Autodesk Fusion 360 part; units mm, degrees
(part 2 of 4)
  spline S203 degree 2 poles (-3.5776, -2.4093) (-3.5776, -2.6712) (-3.7686, -2.854) knots 0 0 0 1 1 1
  spline S204 degree 2 poles (-3.7686, -2.854) (-3.9596, -3.0355) (-4.2515, -3.0355) knots 0 0 0 1 1 1
  spline S205 degree 2 poles (-4.2515, -3.0355) (-4.5148, -3.0355) (-4.6894, -2.8786) knots 0 0 0 1 1 1
  spline S206 degree 2 poles (-4.6894, -2.8786) (-4.8627, -2.7217) (-4.8872, -2.472) knots 0 0 0 1 1 1
  line L129 (-3.2351, -3) -> (-3.2351, -1)
  line L130 (-3.2351, -1) -> (-2.5462, -1)
  spline S207 degree 2 poles (-2.5462, -1) (-2.3129, -1) (-2.1901, -1.0286) knots 0 0 0 1 1 1
  spline S208 degree 2 poles (-2.1901, -1.0286) (-2.0182, -1.0682) (-1.8968, -1.1719) knots 0 0 0 1 1 1
  spline S209 degree 2 poles (-1.8968, -1.1719) (-1.7385, -1.3056) (-1.6608, -1.5143) knots 0 0 0 1 1 1
  spline S210 degree 2 poles (-1.6608, -1.5143) (-1.5817, -1.7217) (-1.5817, -1.9891) knots 0 0 0 1 1 1
  spline S211 degree 2 poles (-1.5817, -1.9891) (-1.5817, -2.2169) (-1.6349, -2.3929) knots 0 0 0 1 1 1
  spline S212 degree 2 poles (-1.6349, -2.3929) (-1.6881, -2.5689) (-1.7713, -2.6849) knots 0 0 0 1 1 1
  spline S213 degree 2 poles (-1.7713, -2.6849) (-1.8545, -2.7995) (-1.9541, -2.8663) knots 0 0 0 1 1 1
  spline S214 degree 2 poles (-1.9541, -2.8663) (-2.0523, -2.9318) (-2.1928, -2.9659) knots 0 0 0 1 1 1
  spline S215 degree 2 poles (-2.1928, -2.9659) (-2.332, -3) (-2.5134, -3) knots 0 0 0 1 1 1
  line L131 (-2.5134, -3) -> (-3.2351, -3)
  line L132 (-2.9705, -2.764) -> (-2.5435, -2.764)
  spline S216 degree 2 poles (-2.5435, -2.764) (-2.3456, -2.764) (-2.2338, -2.7271) knots 0 0 0 1 1 1
  spline S217 degree 2 poles (-2.2338, -2.7271) (-2.1205, -2.6903) (-2.0537, -2.6235) knots 0 0 0 1 1 1
  spline S218 degree 2 poles (-2.0537, -2.6235) (-1.9596, -2.5293) (-1.9077, -2.3711) knots 0 0 0 1 1 1
  spline S219 degree 2 poles (-1.9077, -2.3711) (-1.8545, -2.2115) (-1.8545, -1.985) knots 0 0 0 1 1 1
  spline S220 degree 2 poles (-1.8545, -1.985) (-1.8545, -1.6712) (-1.9582, -1.5034) knots 0 0 0 1 1 1
  spline S221 degree 2 poles (-1.9582, -1.5034) (-2.0605, -1.3342) (-2.2078, -1.2769) knots 0 0 0 1 1 1
  spline S222 degree 2 poles (-2.2078, -1.2769) (-2.3143, -1.236) (-2.5503, -1.236) knots 0 0 0 1 1 1
  line L133 (-2.5503, -1.236) -> (-2.9705, -1.236)
  line L134 (-2.9705, -1.236) -> (-2.9705, -2.764)
  line L135 (-0.5298, -3) -> (-0.5298, -2.5211)
  line L136 (-0.5298, -2.5211) -> (-1.3975, -2.5211)
  line L137 (-1.3975, -2.5211) -> (-1.3975, -2.296)
  line L138 (-1.3975, -2.296) -> (-0.4848, -1)
  line L139 (-0.4848, -1) -> (-0.2842, -1)
  line L140 (-0.2842, -1) -> (-0.2842, -2.296)
  line L141 (-0.2842, -2.296) -> (-0.0141, -2.296)
  line L142 (-0.0141, -2.296) -> (-0.0141, -2.5211)
  line L143 (-0.0141, -2.5211) -> (-0.2842, -2.5211)
  line L144 (-0.2842, -2.5211) -> (-0.2842, -3)
  line L145 (-0.2842, -3) -> (-0.5298, -3)
  line L146 (-0.5298, -2.296) -> (-0.5298, -1.3943)
  line L147 (-0.5298, -1.3943) -> (-1.156, -2.296)
  line L148 (-1.156, -2.296) -> (-0.5298, -2.296)
  line L149 (0.2096, -2.3997) -> (0.2096, -2.1528)
  line L150 (0.2096, -2.1528) -> (0.964, -2.1528)
  line L151 (0.964, -2.1528) -> (0.964, -2.3997)
  line L152 (0.964, -2.3997) -> (0.2096, -2.3997)
  line L153 (1.1769, -2.3574) -> (1.4265, -2.3356)
  spline S223 degree 2 poles (1.4265, -2.3356) (1.4443, -2.4857) (1.5084, -2.5825) knots 0 0 0 1 1 1
  spline S224 degree 2 poles (1.5084, -2.5825) (1.5739, -2.678) (1.7103, -2.7381) knots 0 0 0 1 1 1
  spline S225 degree 2 poles (1.7103, -2.7381) (1.8467, -2.7967) (2.0173, -2.7967) knots 0 0 0 1 1 1
  spline S226 degree 2 poles (2.0173, -2.7967) (2.1687, -2.7967) (2.2847, -2.7517) knots 0 0 0 1 1 1
  spline S227 degree 2 poles (2.2847, -2.7517) (2.4006, -2.7067) (2.4565, -2.6289) knots 0 0 0 1 1 1
  spline S228 degree 2 poles (2.4565, -2.6289) (2.5138, -2.5498) (2.5138, -2.457) knots 0 0 0 1 1 1
  spline S229 degree 2 poles (2.5138, -2.457) (2.5138, -2.3629) (2.4593, -2.2933) knots 0 0 0 1 1 1
  spline S230 degree 2 poles (2.4593, -2.2933) (2.4047, -2.2224) (2.2792, -2.1746) knots 0 0 0 1 1 1
  spline S231 degree 2 poles (2.2792, -2.1746) (2.1987, -2.1432) (1.9231, -2.0778) knots 0 0 0 1 1 1
  spline S232 degree 2 poles (1.9231, -2.0778) (1.6475, -2.0109) (1.537, -1.9523) knots 0 0 0 1 1 1
  spline S233 degree 2 poles (1.537, -1.9523) (1.3938, -1.8772) (1.3229, -1.7667) knots 0 0 0 1 1 1
  spline S234 degree 2 poles (1.3229, -1.7667) (1.2533, -1.6548) (1.2533, -1.5171) knots 0 0 0 1 1 1
  spline S235 degree 2 poles (1.2533, -1.5171) (1.2533, -1.3656) (1.3392, -1.2347) knots 0 0 0 1 1 1
  spline S236 degree 2 poles (1.3392, -1.2347) (1.4252, -1.1023) (1.5902, -1.0341) knots 0 0 0 1 1 1
  spline S237 degree 2 poles (1.5902, -1.0341) (1.7553, -0.9659) (1.9572, -0.9659) knots 0 0 0 1 1 1
  spline S238 degree 2 poles (1.9572, -0.9659) (2.1796, -0.9659) (2.3488, -1.0382) knots 0 0 0 1 1 1
  spline S239 degree 2 poles (2.3488, -1.0382) (2.5193, -1.1091) (2.6107, -1.2483) knots 0 0 0 1 1 1
  spline S240 degree 2 poles (2.6107, -1.2483) (2.7021, -1.3874) (2.7089, -1.5634) knots 0 0 0 1 1 1
  line L154 (2.7089, -1.5634) -> (2.4552, -1.5825)
  spline S241 degree 2 poles (2.4552, -1.5825) (2.4347, -1.3929) (2.316, -1.296) knots 0 0 0 1 1 1
  spline S242 degree 2 poles (2.316, -1.296) (2.1987, -1.1992) (1.9681, -1.1992) knots 0 0 0 1 1 1
  spline S243 degree 2 poles (1.9681, -1.1992) (1.728, -1.1992) (1.6175, -1.2879) knots 0 0 0 1 1 1
  spline S244 degree 2 poles (1.6175, -1.2879) (1.5084, -1.3752) (1.5084, -1.4993) knots 0 0 0 1 1 1
  spline S245 degree 2 poles (1.5084, -1.4993) (1.5084, -1.6071) (1.5862, -1.6767) knots 0 0 0 1 1 1
  spline S246 degree 2 poles (1.5862, -1.6767) (1.6626, -1.7462) (1.9845, -1.8199) knots 0 0 0 1 1 1
  spline S247 degree 2 poles (1.9845, -1.8199) (2.3078, -1.8922) (2.4279, -1.9468) knots 0 0 0 1 1 1
  spline S248 degree 2 poles (2.4279, -1.9468) (2.6025, -2.0273) (2.6857, -2.1514) knots 0 0 0 1 1 1
  spline S249 degree 2 poles (2.6857, -2.1514) (2.769, -2.2742) (2.769, -2.4352) knots 0 0 0 1 1 1
  spline S250 degree 2 poles (2.769, -2.4352) (2.769, -2.5948) (2.6776, -2.7367) knots 0 0 0 1 1 1
  spline S251 degree 2 poles (2.6776, -2.7367) (2.5862, -2.8772) (2.4143, -2.9563) knots 0 0 0 1 1 1
  spline S252 degree 2 poles (2.4143, -2.9563) (2.2437, -3.0341) (2.0295, -3.0341) knots 0 0 0 1 1 1
  spline S253 degree 2 poles (2.0295, -3.0341) (1.758, -3.0341) (1.5739, -2.955) knots 0 0 0 1 1 1
  spline S254 degree 2 poles (1.5739, -2.955) (1.3911, -2.8759) (1.286, -2.7176) knots 0 0 0 1 1 1
  spline S255 degree 2 poles (1.286, -2.7176) (1.1823, -2.558) (1.1769, -2.3574) knots 0 0 0 1 1 1
  line L155 (3.1305, -3) -> (3.1305, -1)
  line L156 (3.1305, -1) -> (3.8194, -1)
  spline S256 degree 2 poles (3.8194, -1) (4.0527, -1) (4.1755, -1.0286) knots 0 0 0 1 1 1
  spline S257 degree 2 poles (4.1755, -1.0286) (4.3474, -1.0682) (4.4688, -1.1719) knots 0 0 0 1 1 1
  spline S258 degree 2 poles (4.4688, -1.1719) (4.6271, -1.3056) (4.7048, -1.5143) knots 0 0 0 1 1 1
  spline S259 degree 2 poles (4.7048, -1.5143) (4.784, -1.7217) (4.784, -1.9891) knots 0 0 0 1 1 1
  spline S260 degree 2 poles (4.784, -1.9891) (4.784, -2.2169) (4.7308, -2.3929) knots 0 0 0 1 1 1
  spline S261 degree 2 poles (4.7308, -2.3929) (4.6776, -2.5689) (4.5943, -2.6849) knots 0 0 0 1 1 1
  spline S262 degree 2 poles (4.5943, -2.6849) (4.5111, -2.7995) (4.4115, -2.8663) knots 0 0 0 1 1 1
  spline S263 degree 2 poles (4.4115, -2.8663) (4.3133, -2.9318) (4.1728, -2.9659) knots 0 0 0 1 1 1
  spline S264 degree 2 poles (4.1728, -2.9659) (4.0336, -3) (3.8522, -3) knots 0 0 0 1 1 1
  line L157 (3.8522, -3) -> (3.1305, -3)
  line L158 (3.3952, -2.764) -> (3.8222, -2.764)
  spline S265 degree 2 poles (3.8222, -2.764) (4.02, -2.764) (4.1319, -2.7271) knots 0 0 0 1 1 1
  spline S266 degree 2 poles (4.1319, -2.7271) (4.2451, -2.6903) (4.3119, -2.6235) knots 0 0 0 1 1 1
  spline S267 degree 2 poles (4.3119, -2.6235) (4.4061, -2.5293) (4.4579, -2.3711) knots 0 0 0 1 1 1
  spline S268 degree 2 poles (4.4579, -2.3711) (4.5111, -2.2115) (4.5111, -1.985) knots 0 0 0 1 1 1
  spline S269 degree 2 poles (4.5111, -1.985) (4.5111, -1.6712) (4.4074, -1.5034) knots 0 0 0 1 1 1
  spline S270 degree 2 poles (4.4074, -1.5034) (4.3051, -1.3342) (4.1578, -1.2769) knots 0 0 0 1 1 1
  spline S271 degree 2 poles (4.1578, -1.2769) (4.0514, -1.236) (3.8153, -1.236) knots 0 0 0 1 1 1
  line L159 (3.8153, -1.236) -> (3.3952, -1.236)
  line L160 (3.3952, -1.236) -> (3.3952, -2.764)
  spline S272 degree 2 poles (5.5862, -3.588) (5.3829, -3.3315) (5.2424, -2.9877) knots 0 0 0 1 1 1
  spline S273 degree 2 poles (5.2424, -2.9877) (5.1018, -2.6439) (5.1018, -2.2756) knots 0 0 0 1 1 1
  spline S274 degree 2 poles (5.1018, -2.2756) (5.1018, -1.9509) (5.2069, -1.6535) knots 0 0 0 1 1 1
  spline S275 degree 2 poles (5.2069, -1.6535) (5.3297, -1.3083) (5.5862, -0.9659) knots 0 0 0 1 1 1
  line L161 (5.5862, -0.9659) -> (5.7621, -0.9659)
  spline S276 degree 2 poles (5.7621, -0.9659) (5.5971, -1.2497) (5.5439, -1.3711) knots 0 0 0 1 1 1
  spline S277 degree 2 poles (5.5439, -1.3711) (5.4606, -1.5593) (5.4129, -1.764) knots 0 0 0 1 1 1
  spline S278 degree 2 poles (5.4129, -1.764) (5.3542, -2.0191) (5.3542, -2.2769) knots 0 0 0 1 1 1
  spline S279 degree 2 poles (5.3542, -2.2769) (5.3542, -2.9332) (5.7621, -3.588) knots 0 0 0 1 1 1
  line L162 (5.7621, -3.588) -> (5.5862, -3.588)
  line L163 (6.904, -3) -> (6.6585, -3)
  line L164 (6.6585, -3) -> (6.6585, -1.4352)
  spline S280 degree 2 poles (6.6585, -1.4352) (6.5698, -1.5198) (6.4252, -1.6044) knots 0 0 0 1 1 1
  spline S281 degree 2 poles (6.4252, -1.6044) (6.2819, -1.6889) (6.1673, -1.7312) knots 0 0 0 1 1 1
  line L165 (6.1673, -1.7312) -> (6.1673, -1.4939)
  spline S282 degree 2 poles (6.1673, -1.4939) (6.3733, -1.397) (6.5275, -1.2592) knots 0 0 0 1 1 1
  spline S283 degree 2 poles (6.5275, -1.2592) (6.6816, -1.1214) (6.7458, -0.9918) knots 0 0 0 1 1 1
  line L166 (6.7458, -0.9918) -> (6.904, -0.9918)
  line L167 (6.904, -0.9918) -> (6.904, -3)
  line L168 (7.5329, -2.4761) -> (7.7908, -2.4543)
  spline S284 degree 2 poles (7.7908, -2.4543) (7.8194, -2.6426) (7.9231, -2.7381) knots 0 0 0 1 1 1
  spline S285 degree 2 poles (7.9231, -2.7381) (8.0282, -2.8322) (8.1755, -2.8322) knots 0 0 0 1 1 1
  spline S286 degree 2 poles (8.1755, -2.8322) (8.3529, -2.8322) (8.4756, -2.6985) knots 0 0 0 1 1 1
  spline S287 degree 2 poles (8.4756, -2.6985) (8.5984, -2.5648) (8.5984, -2.3438) knots 0 0 0 1 1 1
  spline S288 degree 2 poles (8.5984, -2.3438) (8.5984, -2.1337) (8.4797, -2.0123) knots 0 0 0 1 1 1
  spline S289 degree 2 poles (8.4797, -2.0123) (8.3624, -1.8909) (8.1714, -1.8909) knots 0 0 0 1 1 1
  spline S290 degree 2 poles (8.1714, -1.8909) (8.0527, -1.8909) (7.9572, -1.9454) knots 0 0 0 1 1 1
  spline S291 degree 2 poles (7.9572, -1.9454) (7.8617, -1.9986) (7.8072, -2.0846) knots 0 0 0 1 1 1
  line L169 (7.8072, -2.0846) -> (7.5766, -2.0546)
  line L170 (7.5766, -2.0546) -> (7.7703, -1.0273)
  line L171 (7.7703, -1.0273) -> (8.7649, -1.0273)
  line L172 (8.7649, -1.0273) -> (8.7649, -1.2619)
  line L173 (8.7649, -1.2619) -> (7.9668, -1.2619)
  line L174 (7.9668, -1.2619) -> (7.859, -1.7995)
  spline S292 degree 2 poles (7.859, -1.7995) (8.0391, -1.6739) (8.2369, -1.6739) knots 0 0 0 1 1 1
  spline S293 degree 2 poles (8.2369, -1.6739) (8.4988, -1.6739) (8.6789, -1.8554) knots 0 0 0 1 1 1
  spline S294 degree 2 poles (8.6789, -1.8554) (8.859, -2.0368) (8.859, -2.322) knots 0 0 0 1 1 1
  spline S295 degree 2 poles (8.859, -2.322) (8.859, -2.5935) (8.7007, -2.7913) knots 0 0 0 1 1 1
  spline S296 degree 2 poles (8.7007, -2.7913) (8.5084, -3.0341) (8.1755, -3.0341) knots 0 0 0 1 1 1
  spline S297 degree 2 poles (8.1755, -3.0341) (7.9027, -3.0341) (7.7294, -2.8813) knots 0 0 0 1 1 1
  spline S298 degree 2 poles (7.7294, -2.8813) (7.5575, -2.7285) (7.5329, -2.4761) knots 0 0 0 1 1 1
  line L175 (9.1032, -1.2619) -> (9.1032, -1.0259)
  line L176 (9.1032, -1.0259) -> (10.3979, -1.0259)
  line L177 (10.3979, -1.0259) -> (10.3979, -1.2169)
  spline S299 degree 2 poles (10.3979, -1.2169) (10.2069, -1.4202) (10.0186, -1.7572) knots 0 0 0 1 1 1
  spline S300 degree 2 poles (10.0186, -1.7572) (9.8317, -2.0941) (9.7294, -2.4502) knots 0 0 0 1 1 1
  spline S301 degree 2 poles (9.7294, -2.4502) (9.6557, -2.7012) (9.6353, -3) knots 0 0 0 1 1 1
  line L178 (9.6353, -3) -> (9.3829, -3)
  spline S302 degree 2 poles (9.3829, -3) (9.387, -2.764) (9.4756, -2.4297) knots 0 0 0 1 1 1
  spline S303 degree 2 poles (9.4756, -2.4297) (9.5643, -2.0955) (9.7294, -1.7858) knots 0 0 0 1 1 1
  spline S304 degree 2 poles (9.7294, -1.7858) (9.8958, -1.4748) (10.0827, -1.2619) knots 0 0 0 1 1 1
  line L179 (10.0827, -1.2619) -> (9.1032, -1.2619)
  line L180 (10.8699, -3.588) -> (10.6939, -3.588)
  spline S305 degree 2 poles (10.6939, -3.588) (11.1018, -2.9332) (11.1018, -2.2769) knots 0 0 0 1 1 1
  spline S306 degree 2 poles (11.1018, -2.2769) (11.1018, -2.0205) (11.0432, -1.7681) knots 0 0 0 1 1 1
  spline S307 degree 2 poles (11.0432, -1.7681) (10.9968, -1.5634) (10.9136, -1.3752) knots 0 0 0 1 1 1
  spline S308 degree 2 poles (10.9136, -1.3752) (10.8604, -1.2524) (10.6939, -0.9659) knots 0 0 0 1 1 1
  line L181 (10.6939, -0.9659) -> (10.8699, -0.9659)
  spline S309 degree 2 poles (10.8699, -0.9659) (11.1264, -1.3083) (11.2492, -1.6535) knots 0 0 0 1 1 1
  spline S310 degree 2 poles (11.2492, -1.6535) (11.3542, -1.9509) (11.3542, -2.2756) knots 0 0 0 1 1 1
  spline S311 degree 2 poles (11.3542, -2.2756) (11.3542, -2.6439) (11.2123, -2.9877) knots 0 0 0 1 1 1
  spline S312 degree 2 poles (11.2123, -2.9877) (11.0718, -3.3315) (10.8699, -3.588) knots 0 0 0 1 1 1
  spline S313 degree 2 poles (-11.8245, 0.9689) (-11.8245, 1.5664) (-11.5036, 1.9037) knots 0 0 0 1 1 1
  spline S314 degree 2 poles (-11.5036, 1.9037) (-11.1827, 2.2426) (-10.6752, 2.2426) knots 0 0 0 1 1 1
  spline S315 degree 2 poles (-10.6752, 2.2426) (-10.3429, 2.2426) (-10.0761, 2.0838) knots 0 0 0 1 1 1
  spline S316 degree 2 poles (-10.0761, 2.0838) (-9.8092, 1.925) (-9.6701, 1.6401) knots 0 0 0 1 1 1
  spline S317 degree 2 poles (-9.6701, 1.6401) (-9.5293, 1.3569) (-9.5293, 0.9967) knots 0 0 0 1 1 1
  spline S318 degree 2 poles (-9.5293, 0.9967) (-9.5293, 0.6317) (-9.6766, 0.3435) knots 0 0 0 1 1 1
  spline S319 degree 2 poles (-9.6766, 0.3435) (-9.8239, 0.0554) (-10.0941, -0.0936) knots 0 0 0 1 1 1
  spline S320 degree 2 poles (-10.0941, -0.0936) (-10.3642, -0.2409) (-10.6769, -0.2409) knots 0 0 0 1 1 1
  spline S321 degree 2 poles (-10.6769, -0.2409) (-11.0158, -0.2409) (-11.2826, -0.0772) knots 0 0 0 1 1 1
  spline S322 degree 2 poles (-11.2826, -0.0772) (-11.5495, 0.0865) (-11.687, 0.3697) knots 0 0 0 1 1 1
  spline S323 degree 2 poles (-11.687, 0.3697) (-11.8245, 0.6529) (-11.8245, 0.9689) knots 0 0 0 1 1 1
  spline S324 degree 2 poles (-11.4971, 0.964) (-11.4971, 0.5302) (-11.2646, 0.2797) knots 0 0 0 1 1 1
  spline S325 degree 2 poles (-11.2646, 0.2797) (-11.0305, 0.0308) (-10.6785, 0.0308) knots 0 0 0 1 1 1
  spline S326 degree 2 poles (-10.6785, 0.0308) (-10.32, 0.0308) (-10.0892, 0.2829) knots 0 0 0 1 1 1
  spline S327 degree 2 poles (-10.0892, 0.2829) (-9.8567, 0.5351) (-9.8567, 0.9984) knots 0 0 0 1 1 1
  spline S328 degree 2 poles (-9.8567, 0.9984) (-9.8567, 1.2914) (-9.9565, 1.5091) knots 0 0 0 1 1 1
  spline S329 degree 2 poles (-9.9565, 1.5091) (-10.0548, 1.7285) (-10.2463, 1.848) knots 0 0 0 1 1 1
  spline S330 degree 2 poles (-10.2463, 1.848) (-10.4362, 1.9692) (-10.6736, 1.9692) knots 0 0 0 1 1 1
  spline S331 degree 2 poles (-10.6736, 1.9692) (-11.0108, 1.9692) (-11.2548, 1.7367) knots 0 0 0 1 1 1
  spline S332 degree 2 poles (-11.2548, 1.7367) (-11.4971, 1.5059) (-11.4971, 0.964) knots 0 0 0 1 1 1
  line L182 (-8.8816, -0.2) -> (-8.8816, 2.2)
  line L183 (-8.8816, 2.2) -> (-7.9812, 2.2)
  spline S333 degree 2 poles (-7.9812, 2.2) (-7.7062, 2.2) (-7.5408, 2.1263) knots 0 0 0 1 1 1
  spline S334 degree 2 poles (-7.5408, 2.1263) (-7.3738, 2.0543) (-7.2805, 1.902) knots 0 0 0 1 1 1
  spline S335 degree 2 poles (-7.2805, 1.902) (-7.1856, 1.7514) (-7.1856, 1.5861) knots 0 0 0 1 1 1
  spline S336 degree 2 poles (-7.1856, 1.5861) (-7.1856, 1.4322) (-7.2691, 1.2963) knots 0 0 0 1 1 1
  spline S337 degree 2 poles (-7.2691, 1.2963) (-7.3526, 1.1604) (-7.5212, 1.0769) knots 0 0 0 1 1 1
  spline S338 degree 2 poles (-7.5212, 1.0769) (-7.3035, 1.0131) (-7.1872, 0.8592) knots 0 0 0 1 1 1
  spline S339 degree 2 poles (-7.1872, 0.8592) (-7.0693, 0.7053) (-7.0693, 0.4958) knots 0 0 0 1 1 1
  spline S340 degree 2 poles (-7.0693, 0.4958) (-7.0693, 0.3271) (-7.1414, 0.1814) knots 0 0 0 1 1 1
  spline S341 degree 2 poles (-7.1414, 0.1814) (-7.2118, 0.0374) (-7.3165, -0.0412) knots 0 0 0 1 1 1
  spline S342 degree 2 poles (-7.3165, -0.0412) (-7.4213, -0.1198) (-7.5801, -0.1607) knots 0 0 0 1 1 1
  spline S343 degree 2 poles (-7.5801, -0.1607) (-7.7373, -0.2) (-7.9665, -0.2) knots 0 0 0 1 1 1
  line L184 (-7.9665, -0.2) -> (-8.8816, -0.2)
  line L185 (-8.564, 1.1915) -> (-8.0451, 1.1915)
  spline S344 degree 2 poles (-8.0451, 1.1915) (-7.8339, 1.1915) (-7.7422, 1.2194) knots 0 0 0 1 1 1
  spline S345 degree 2 poles (-7.7422, 1.2194) (-7.6211, 1.2554) (-7.5605, 1.3389) knots 0 0 0 1 1 1
  spline S346 degree 2 poles (-7.5605, 1.3389) (-7.4983, 1.4224) (-7.4983, 1.5484) knots 0 0 0 1 1 1
  spline S347 degree 2 poles (-7.4983, 1.5484) (-7.4983, 1.6679) (-7.5556, 1.758) knots 0 0 0 1 1 1
  spline S348 degree 2 poles (-7.5556, 1.758) (-7.6129, 1.8497) (-7.7193, 1.8824) knots 0 0 0 1 1 1
  spline S349 degree 2 poles (-7.7193, 1.8824) (-7.8257, 1.9168) (-8.0844, 1.9168) knots 0 0 0 1 1 1
  line L186 (-8.0844, 1.9168) -> (-8.564, 1.9168)
  line L187 (-8.564, 1.9168) -> (-8.564, 1.1915)
  line L188 (-8.564, 0.0832) -> (-7.9665, 0.0832)
  spline S350 degree 2 poles (-7.9665, 0.0832) (-7.8126, 0.0832) (-7.7504, 0.0947) knots 0 0 0 1 1 1
  spline S351 degree 2 poles (-7.7504, 0.0947) (-7.6407, 0.1143) (-7.567, 0.1602) knots 0 0 0 1 1 1
  spline S352 degree 2 poles (-7.567, 0.1602) (-7.4934, 0.206) (-7.4459, 0.2928) knots 0 0 0 1 1 1
  spline S353 degree 2 poles (-7.4459, 0.2928) (-7.3984, 0.3812) (-7.3984, 0.4958) knots 0 0 0 1 1 1
  spline S354 degree 2 poles (-7.3984, 0.4958) (-7.3984, 0.63) (-7.4672, 0.7282) knots 0 0 0 1 1 1
  spline S355 degree 2 poles (-7.4672, 0.7282) (-7.5359, 0.8281) (-7.6587, 0.8674) knots 0 0 0 1 1 1
  spline S356 degree 2 poles (-7.6587, 0.8674) (-7.7799, 0.9083) (-8.009, 0.9083) knots 0 0 0 1 1 1
  line L189 (-8.009, 0.9083) -> (-8.564, 0.9083)
  line L190 (-8.564, 0.9083) -> (-8.564, 0.0832)
  line L191 (-6.4888, 0.5711) -> (-6.1892, 0.5973)
  spline S357 degree 2 poles (-6.1892, 0.5973) (-6.168, 0.4172) (-6.091, 0.301) knots 0 0 0 1 1 1
  spline S358 degree 2 poles (-6.091, 0.301) (-6.0124, 0.1864) (-5.8487, 0.1143) knots 0 0 0 1 1 1
  spline S359 degree 2 poles (-5.8487, 0.1143) (-5.685, 0.0439) (-5.4804, 0.0439) knots 0 0 0 1 1 1
  spline S360 degree 2 poles (-5.4804, 0.0439) (-5.2987, 0.0439) (-5.1595, 0.098) knots 0 0 0 1 1 1
  spline S361 degree 2 poles (-5.1595, 0.098) (-5.0203, 0.152) (-4.9532, 0.2453) knots 0 0 0 1 1 1
  spline S362 degree 2 poles (-4.9532, 0.2453) (-4.8845, 0.3402) (-4.8845, 0.4516) knots 0 0 0 1 1 1
  spline S363 degree 2 poles (-4.8845, 0.4516) (-4.8845, 0.5645) (-4.9499, 0.648) knots 0 0 0 1 1 1
  spline S364 degree 2 poles (-4.9499, 0.648) (-5.0154, 0.7332) (-5.166, 0.7905) knots 0 0 0 1 1 1
  spline S365 degree 2 poles (-5.166, 0.7905) (-5.2626, 0.8281) (-5.5933, 0.9067) knots 0 0 0 1 1 1
  spline S366 degree 2 poles (-5.5933, 0.9067) (-5.924, 0.9869) (-6.0566, 1.0573) knots 0 0 0 1 1 1
  spline S367 degree 2 poles (-6.0566, 1.0573) (-6.2285, 1.1473) (-6.3137, 1.2799) knots 0 0 0 1 1 1
  spline S368 degree 2 poles (-6.3137, 1.2799) (-6.3971, 1.4142) (-6.3971, 1.5795) knots 0 0 0 1 1 1
  spline S369 degree 2 poles (-6.3971, 1.5795) (-6.3971, 1.7613) (-6.294, 1.9184) knots 0 0 0 1 1 1
  spline S370 degree 2 poles (-6.294, 1.9184) (-6.1909, 2.0772) (-5.9928, 2.1591) knots 0 0 0 1 1 1
  spline S371 degree 2 poles (-5.9928, 2.1591) (-5.7947, 2.2409) (-5.5524, 2.2409) knots 0 0 0 1 1 1
  spline S372 degree 2 poles (-5.5524, 2.2409) (-5.2856, 2.2409) (-5.0826, 2.1542) knots 0 0 0 1 1 1
  spline S373 degree 2 poles (-5.0826, 2.1542) (-4.8779, 2.069) (-4.7682, 1.902) knots 0 0 0 1 1 1
  spline S374 degree 2 poles (-4.7682, 1.902) (-4.6585, 1.7351) (-4.6504, 1.5239) knots 0 0 0 1 1 1
  line L192 (-4.6504, 1.5239) -> (-4.9549, 1.501)
  spline S375 degree 2 poles (-4.9549, 1.501) (-4.9794, 1.7285) (-5.1218, 1.8447) knots 0 0 0 1 1 1
  spline S376 degree 2 poles (-5.1218, 1.8447) (-5.2626, 1.961) (-5.5393, 1.961) knots 0 0 0 1 1 1
  spline S377 degree 2 poles (-5.5393, 1.961) (-5.8274, 1.961) (-5.96, 1.8546) knots 0 0 0 1 1 1
  spline S378 degree 2 poles (-5.96, 1.8546) (-6.091, 1.7498) (-6.091, 1.6008) knots 0 0 0 1 1 1
  spline S379 degree 2 poles (-6.091, 1.6008) (-6.091, 1.4715) (-5.9977, 1.388) knots 0 0 0 1 1 1
  spline S380 degree 2 poles (-5.9977, 1.388) (-5.906, 1.3045) (-5.5197, 1.2161) knots 0 0 0 1 1 1
  spline S381 degree 2 poles (-5.5197, 1.2161) (-5.1317, 1.1293) (-4.9876, 1.0638) knots 0 0 0 1 1 1
  spline S382 degree 2 poles (-4.9876, 1.0638) (-4.778, 0.9673) (-4.6782, 0.8183) knots 0 0 0 1 1 1
  spline S383 degree 2 poles (-4.6782, 0.8183) (-4.5783, 0.6709) (-4.5783, 0.4778) knots 0 0 0 1 1 1
  spline S384 degree 2 poles (-4.5783, 0.4778) (-4.5783, 0.2862) (-4.688, 0.116) knots 0 0 0 1 1 1
  spline S385 degree 2 poles (-4.688, 0.116) (-4.7977, -0.0527) (-5.004, -0.1476) knots 0 0 0 1 1 1
  spline S386 degree 2 poles (-5.004, -0.1476) (-5.2086, -0.2409) (-5.4656, -0.2409) knots 0 0 0 1 1 1
  spline S387 degree 2 poles (-5.4656, -0.2409) (-5.7914, -0.2409) (-6.0124, -0.146) knots 0 0 0 1 1 1
  spline S388 degree 2 poles (-6.0124, -0.146) (-6.2318, -0.051) (-6.3579, 0.1389) knots 0 0 0 1 1 1
  spline S389 degree 2 poles (-6.3579, 0.1389) (-6.4823, 0.3304) (-6.4888, 0.5711) knots 0 0 0 1 1 1
  line L193 (-4.1566, -0.2) -> (-3.2349, 2.2)
  line L194 (-3.2349, 2.2) -> (-2.8928, 2.2)
  line L195 (-2.8928, 2.2) -> (-1.9105, -0.2)
  line L196 (-1.9105, -0.2) -> (-2.2723, -0.2)
  line L197 (-2.2723, -0.2) -> (-2.5522, 0.5269)
  line L198 (-2.5522, 0.5269) -> (-3.5558, 0.5269)
  line L199 (-3.5558, 0.5269) -> (-3.8194, -0.2)
  line L200 (-3.8194, -0.2) -> (-4.1566, -0.2)
  line L201 (-3.4641, 0.7855) -> (-2.6505, 0.7855)
  line L202 (-2.6505, 0.7855) -> (-2.9009, 1.4502)
  spline S390 degree 2 poles (-2.9009, 1.4502) (-3.0155, 1.7531) (-3.0712, 1.9479) knots 0 0 0 1 1 1
  spline S391 degree 2 poles (-3.0712, 1.9479) (-3.117, 1.7171) (-3.2005, 1.4895) knots 0 0 0 1 1 1
  line L203 (-3.2005, 1.4895) -> (-3.4641, 0.7855)
  line L204 (-1.5575, 0.5203) -> (-1.5575, 0.8166)
  line L205 (-1.5575, 0.8166) -> (-0.6522, 0.8166)
  line L206 (-0.6522, 0.8166) -> (-0.6522, 0.5203)
  line L207 (-0.6522, 0.5203) -> (-1.5575, 0.5203)
  line L208 (-0.0504, -0.2) -> (-0.0504, 2.2)
  line L209 (-0.0504, 2.2) -> (0.2672, 2.2)
  line L210 (0.2672, 2.2) -> (0.2672, 0.0832)
  line L211 (0.2672, 0.0832) -> (1.4492, 0.0832)
  line L212 (1.4492, 0.0832) -> (1.4492, -0.2)
  line L213 (1.4492, -0.2) -> (-0.0504, -0.2)
  line L214 (2.0886, -0.2) -> (2.0886, 2.2)
  line L215 (2.0886, 2.2) -> (2.4062, 2.2)
  line L216 (2.4062, 2.2) -> (2.4062, 1.2145)
  line L217 (2.4062, 1.2145) -> (3.6537, 1.2145)
  line L218 (3.6537, 1.2145) -> (3.6537, 2.2)
  line L219 (3.6537, 2.2) -> (3.9713, 2.2)
  line L220 (3.9713, 2.2) -> (3.9713, -0.2)
  line L221 (3.9713, -0.2) -> (3.6537, -0.2)
  line L222 (3.6537, -0.2) -> (3.6537, 0.9312)
  line L223 (3.6537, 0.9312) -> (2.4062, 0.9312)
  line L224 (2.4062, 0.9312) -> (2.4062, -0.2)
  line L225 (2.4062, -0.2) -> (2.0886, -0.2)
  line L226 (4.6435, 0.5711) -> (4.9431, 0.5973)
  spline S392 degree 2 poles (4.9431, 0.5973) (4.9644, 0.4172) (5.0413, 0.301) knots 0 0 0 1 1 1
  spline S393 degree 2 poles (5.0413, 0.301) (5.1199, 0.1864) (5.2836, 0.1143) knots 0 0 0 1 1 1
  spline S394 degree 2 poles (5.2836, 0.1143) (5.4473, 0.0439) (5.652, 0.0439) knots 0 0 0 1 1 1
  spline S395 degree 2 poles (5.652, 0.0439) (5.8337, 0.0439) (5.9728, 0.098) knots 0 0 0 1 1 1
  spline S396 degree 2 poles (5.9728, 0.098) (6.112, 0.152) (6.1791, 0.2453) knots 0 0 0 1 1 1
  spline S397 degree 2 poles (6.1791, 0.2453) (6.2479, 0.3402) (6.2479, 0.4516) knots 0 0 0 1 1 1
  spline S398 degree 2 poles (6.2479, 0.4516) (6.2479, 0.5645) (6.1824, 0.648) knots 0 0 0 1 1 1
  spline S399 degree 2 poles (6.1824, 0.648) (6.1169, 0.7332) (5.9663, 0.7905) knots 0 0 0 1 1 1
  spline S400 degree 2 poles (5.9663, 0.7905) (5.8697, 0.8281) (5.539, 0.9067) knots 0 0 0 1 1 1
  spline S401 degree 2 poles (5.539, 0.9067) (5.2083, 0.9869) (5.0757, 1.0573) knots 0 0 0 1 1 1
  spline S402 degree 2 poles (5.0757, 1.0573) (4.9038, 1.1473) (4.8187, 1.2799) knots 0 0 0 1 1 1
  spline S403 degree 2 poles (4.8187, 1.2799) (4.7352, 1.4142) (4.7352, 1.5795) knots 0 0 0 1 1 1
  spline S404 degree 2 poles (4.7352, 1.5795) (4.7352, 1.7613) (4.8383, 1.9184) knots 0 0 0 1 1 1
  spline S405 degree 2 poles (4.8383, 1.9184) (4.9415, 2.0772) (5.1395, 2.1591) knots 0 0 0 1 1 1
  spline S406 degree 2 poles (5.1395, 2.1591) (5.3376, 2.2409) (5.5799, 2.2409) knots 0 0 0 1 1 1
  spline S407 degree 2 poles (5.5799, 2.2409) (5.8468, 2.2409) (6.0498, 2.1542) knots 0 0 0 1 1 1
  spline S408 degree 2 poles (6.0498, 2.1542) (6.2544, 2.069) (6.3641, 1.902) knots 0 0 0 1 1 1
  spline S409 degree 2 poles (6.3641, 1.902) (6.4738, 1.7351) (6.482, 1.5239) knots 0 0 0 1 1 1
  line L227 (6.482, 1.5239) -> (6.1775, 1.501)
  spline S410 degree 2 poles (6.1775, 1.501) (6.1529, 1.7285) (6.0105, 1.8447) knots 0 0 0 1 1 1
  spline S411 degree 2 poles (6.0105, 1.8447) (5.8697, 1.961) (5.593, 1.961) knots 0 0 0 1 1 1
  spline S412 degree 2 poles (5.593, 1.961) (5.3049, 1.961) (5.1723, 1.8546) knots 0 0 0 1 1 1
  spline S413 degree 2 poles (5.1723, 1.8546) (5.0413, 1.7498) (5.0413, 1.6008) knots 0 0 0 1 1 1
  spline S414 degree 2 poles (5.0413, 1.6008) (5.0413, 1.4715) (5.1346, 1.388) knots 0 0 0 1 1 1
  spline S415 degree 2 poles (5.1346, 1.388) (5.2263, 1.3045) (5.6127, 1.2161) knots 0 0 0 1 1 1
  spline S416 degree 2 poles (5.6127, 1.2161) (6.0007, 1.1293) (6.1447, 1.0638) knots 0 0 0 1 1 1
  spline S417 degree 2 poles (6.1447, 1.0638) (6.3543, 0.9673) (6.4541, 0.8183) knots 0 0 0 1 1 1
  spline S418 degree 2 poles (6.4541, 0.8183) (6.554, 0.6709) (6.554, 0.4778) knots 0 0 0 1 1 1
  spline S419 degree 2 poles (6.554, 0.4778) (6.554, 0.2862) (6.4443, 0.116) knots 0 0 0 1 1 1
  spline S420 degree 2 poles (6.4443, 0.116) (6.3346, -0.0527) (6.1284, -0.1476) knots 0 0 0 1 1 1
  spline S421 degree 2 poles (6.1284, -0.1476) (5.9237, -0.2409) (5.6667, -0.2409) knots 0 0 0 1 1 1
  spline S422 degree 2 poles (5.6667, -0.2409) (5.3409, -0.2409) (5.1199, -0.146) knots 0 0 0 1 1 1
  spline S423 degree 2 poles (5.1199, -0.146) (4.9005, -0.051) (4.7745, 0.1389) knots 0 0 0 1 1 1
  spline S424 degree 2 poles (4.7745, 0.1389) (4.6501, 0.3304) (4.6435, 0.5711) knots 0 0 0 1 1 1
  line L228 (8.2298, -0.2) -> (7.9351, -0.2)
  line L229 (7.9351, -0.2) -> (7.9351, 1.6778)
  spline S425 degree 2 poles (7.9351, 1.6778) (7.8287, 1.5763) (7.6551, 1.4748) knots 0 0 0 1 1 1
  spline S426 degree 2 poles (7.6551, 1.4748) (7.4832, 1.3733) (7.3457, 1.3225) knots 0 0 0 1 1 1
  line L230 (7.3457, 1.3225) -> (7.3457, 1.6074)
  spline S427 degree 2 poles (7.3457, 1.6074) (7.5929, 1.7236) (7.7779, 1.8889) knots 0 0 0 1 1 1
  spline S428 degree 2 poles (7.7779, 1.8889) (7.9629, 2.0543) (8.0398, 2.2098) knots 0 0 0 1 1 1
  line L231 (8.0398, 2.2098) -> (8.2298, 2.2098)
  line L232 (8.2298, 2.2098) -> (8.2298, -0.2)
  line L233 (9.3718, -0.2) -> (9.3718, 2.2)
  line L234 (9.3718, 2.2) -> (10.9909, 2.2)
  line L235 (10.9909, 2.2) -> (10.9909, 1.9168)
  line L236 (10.9909, 1.9168) -> (9.6894, 1.9168)
  line L237 (9.6894, 1.9168) -> (9.6894, 1.1735)
  line L238 (9.6894, 1.1735) -> (10.8157, 1.1735)
  line L239 (10.8157, 1.1735) -> (10.8157, 0.8903)
  line L240 (10.8157, 0.8903) -> (9.6894, 0.8903)
  line L241 (9.6894, 0.8903) -> (9.6894, -0.2)
  line L242 (9.6894, -0.2) -> (9.3718, -0.2)
  spline S429 degree 2 poles (-5.2607, -5.0136) (-5.2607, -4.6589) (-5.1884, -4.4434) knots 0 0 0 1 1 1
  spline S430 degree 2 poles (-5.1884, -4.4434) (-5.1148, -4.2265) (-4.9715, -4.1091) knots 0 0 0 1 1 1
  spline S431 degree 2 poles (-4.9715, -4.1091) (-4.8269, -3.9918) (-4.6086, -3.9918) knots 0 0 0 1 1 1
  spline S432 degree 2 poles (-4.6086, -3.9918) (-4.4476, -3.9918) (-4.3262, -4.0573) knots 0 0 0 1 1 1
  spline S433 degree 2 poles (-4.3262, -4.0573) (-4.2048, -4.1214) (-4.1257, -4.2442) knots 0 0 0 1 1 1
  spline S434 degree 2 poles (-4.1257, -4.2442) (-4.0466, -4.3656) (-4.0015, -4.5416) knots 0 0 0 1 1 1
  spline S435 degree 2 poles (-4.0015, -4.5416) (-3.9565, -4.7162) (-3.9565, -5.0136) knots 0 0 0 1 1 1
  spline S436 degree 2 poles (-3.9565, -5.0136) (-3.9565, -5.3656) (-4.0288, -5.5825) knots 0 0 0 1 1 1
  spline S437 degree 2 poles (-4.0288, -5.5825) (-4.1011, -5.7981) (-4.2457, -5.9168) knots 0 0 0 1 1 1
  spline S438 degree 2 poles (-4.2457, -5.9168) (-4.389, -6.0341) (-4.6086, -6.0341) knots 0 0 0 1 1 1
  spline S439 degree 2 poles (-4.6086, -6.0341) (-4.8979, -6.0341) (-5.0629, -5.8267) knots 0 0 0 1 1 1
  spline S440 degree 2 poles (-5.0629, -5.8267) (-5.2607, -5.5771) (-5.2607, -5.0136) knots 0 0 0 1 1 1
  spline S441 degree 2 poles (-5.0084, -5.0136) (-5.0084, -5.5061) (-4.8938, -5.6698) knots 0 0 0 1 1 1
  spline S442 degree 2 poles (-4.8938, -5.6698) (-4.7778, -5.8322) (-4.6086, -5.8322) knots 0 0 0 1 1 1
  spline S443 degree 2 poles (-4.6086, -5.8322) (-4.4395, -5.8322) (-4.3249, -5.6685) knots 0 0 0 1 1 1
  spline S444 degree 2 poles (-4.3249, -5.6685) (-4.2089, -5.5048) (-4.2089, -5.0136) knots 0 0 0 1 1 1
  spline S445 degree 2 poles (-4.2089, -5.0136) (-4.2089, -4.5198) (-4.3249, -4.3574) knots 0 0 0 1 1 1
  spline S446 degree 2 poles (-4.3249, -4.3574) (-4.4395, -4.1951) (-4.6114, -4.1951) knots 0 0 0 1 1 1
  spline S447 degree 2 poles (-4.6114, -4.1951) (-4.7805, -4.1951) (-4.8815, -4.3383) knots 0 0 0 1 1 1
  spline S448 degree 2 poles (-4.8815, -4.3383) (-5.0084, -4.5211) (-5.0084, -5.0136) knots 0 0 0 1 1 1
  line L243 (-3.5691, -6) -> (-3.5691, -5.7203)
  line L244 (-3.5691, -5.7203) -> (-3.2894, -5.7203)
  line L245 (-3.2894, -5.7203) -> (-3.2894, -6)
  line L246 (-3.2894, -6) -> (-3.5691, -6)
  line L247 (-2.0056, -6) -> (-2.2512, -6)
  line L248 (-2.2512, -6) -> (-2.2512, -4.4352)
  spline S449 degree 2 poles (-2.2512, -4.4352) (-2.3399, -4.5198) (-2.4845, -4.6044) knots 0 0 0 1 1 1
  spline S450 degree 2 poles (-2.4845, -4.6044) (-2.6277, -4.6889) (-2.7423, -4.7312) knots 0 0 0 1 1 1
  line L249 (-2.7423, -4.7312) -> (-2.7423, -4.4939)
  spline S451 degree 2 poles (-2.7423, -4.4939) (-2.5363, -4.397) (-2.3822, -4.2592) knots 0 0 0 1 1 1
  spline S452 degree 2 poles (-2.3822, -4.2592) (-2.228, -4.1214) (-2.1639, -3.9918) knots 0 0 0 1 1 1
  line L250 (-2.1639, -3.9918) -> (-2.0056, -3.9918)
  line L251 (-2.0056, -3.9918) -> (-2.0056, -6)
  line L252 (-1.4968, -6) -> (-0.7287, -4)
  line L253 (-0.7287, -4) -> (-0.4436, -4)
  line L254 (-0.4436, -4) -> (0.375, -6)
  line L255 (0.375, -6) -> (0.0735, -6)
  line L256 (0.0735, -6) -> (-0.1598, -5.3943)
  line L257 (-0.1598, -5.3943) -> (-0.9961, -5.3943)
  line L258 (-0.9961, -5.3943) -> (-1.2157, -6)
  line L259 (-1.2157, -6) -> (-1.4968, -6)
  line L260 (-0.9197, -5.1787) -> (-0.2416, -5.1787)
  line L261 (-0.2416, -5.1787) -> (-0.4504, -4.6248)
  spline S453 degree 2 poles (-0.4504, -4.6248) (-0.5459, -4.3724) (-0.5923, -4.2101) knots 0 0 0 1 1 1
  spline S454 degree 2 poles (-0.5923, -4.2101) (-0.6305, -4.4025) (-0.7, -4.5921) knots 0 0 0 1 1 1
  line L262 (-0.7, -4.5921) -> (-0.9197, -5.1787)
  line L263 (2.596, -5.472) -> (2.8416, -5.4393)
  spline S455 degree 2 poles (2.8416, -5.4393) (2.8839, -5.648) (2.9848, -5.7408) knots 0 0 0 1 1 1
  spline S456 degree 2 poles (2.9848, -5.7408) (3.0871, -5.8322) (3.2331, -5.8322) knots 0 0 0 1 1 1
  spline S457 degree 2 poles (3.2331, -5.8322) (3.4064, -5.8322) (3.5251, -5.7121) knots 0 0 0 1 1 1
  spline S458 degree 2 poles (3.5251, -5.7121) (3.6451, -5.5921) (3.6451, -5.4147) knots 0 0 0 1 1 1
  spline S459 degree 2 poles (3.6451, -5.4147) (3.6451, -5.2456) (3.5346, -5.1364) knots 0 0 0 1 1 1
  spline S460 degree 2 poles (3.5346, -5.1364) (3.4241, -5.0259) (3.2536, -5.0259) knots 0 0 0 1 1 1
  spline S461 degree 2 poles (3.2536, -5.0259) (3.184, -5.0259) (3.0803, -5.0532) knots 0 0 0 1 1 1
  line L264 (3.0803, -5.0532) -> (3.1076, -4.8377)
  spline S462 degree 2 poles (3.1076, -4.8377) (3.1322, -4.8404) (3.1472, -4.8404) knots 0 0 0 1 1 1
  spline S463 degree 2 poles (3.1472, -4.8404) (3.3041, -4.8404) (3.4296, -4.7585) knots 0 0 0 1 1 1
  spline S464 degree 2 poles (3.4296, -4.7585) (3.5551, -4.6767) (3.5551, -4.5061) knots 0 0 0 1 1 1
  spline S465 degree 2 poles (3.5551, -4.5061) (3.5551, -4.3711) (3.4637, -4.2824) knots 0 0 0 1 1 1
  spline S466 degree 2 poles (3.4637, -4.2824) (3.3723, -4.1937) (3.2277, -4.1937) knots 0 0 0 1 1 1
  spline S467 degree 2 poles (3.2277, -4.1937) (3.0844, -4.1937) (2.9889, -4.2838) knots 0 0 0 1 1 1
  spline S468 degree 2 poles (2.9889, -4.2838) (2.8934, -4.3738) (2.8661, -4.5539) knots 0 0 0 1 1 1
  line L265 (2.8661, -4.5539) -> (2.6206, -4.5102)
  spline S469 degree 2 poles (2.6206, -4.5102) (2.6656, -4.2633) (2.8252, -4.1282) knots 0 0 0 1 1 1
  spline S470 degree 2 poles (2.8252, -4.1282) (2.9848, -3.9918) (3.2222, -3.9918) knots 0 0 0 1 1 1
  spline S471 degree 2 poles (3.2222, -3.9918) (3.3859, -3.9918) (3.5237, -4.0628) knots 0 0 0 1 1 1
  spline S472 degree 2 poles (3.5237, -4.0628) (3.6615, -4.1323) (3.7338, -4.2538) knots 0 0 0 1 1 1
  spline S473 degree 2 poles (3.7338, -4.2538) (3.8075, -4.3752) (3.8075, -4.5116) knots 0 0 0 1 1 1
  spline S474 degree 2 poles (3.8075, -4.5116) (3.8075, -4.6412) (3.7379, -4.7476) knots 0 0 0 1 1 1
  spline S475 degree 2 poles (3.7379, -4.7476) (3.6683, -4.854) (3.5319, -4.9168) knots 0 0 0 1 1 1
  spline S476 degree 2 poles (3.5319, -4.9168) (3.7092, -4.9577) (3.8075, -5.0873) knots 0 0 0 1 1 1
  spline S477 degree 2 poles (3.8075, -5.0873) (3.9057, -5.2156) (3.9057, -5.4093) knots 0 0 0 1 1 1
  spline S478 degree 2 poles (3.9057, -5.4093) (3.9057, -5.6712) (3.7147, -5.854) knots 0 0 0 1 1 1
  spline S479 degree 2 poles (3.7147, -5.854) (3.5237, -6.0355) (3.2318, -6.0355) knots 0 0 0 1 1 1
  spline S480 degree 2 poles (3.2318, -6.0355) (2.9685, -6.0355) (2.7938, -5.8786) knots 0 0 0 1 1 1
  spline S481 degree 2 poles (2.7938, -5.8786) (2.6206, -5.7217) (2.596, -5.472) knots 0 0 0 1 1 1
  spline S482 degree 2 poles (4.1485, -5.0136) (4.1485, -4.6589) (4.2208, -4.4434) knots 0 0 0 1 1 1
  spline S483 degree 2 poles (4.2208, -4.4434) (4.2945, -4.2265) (4.4378, -4.1091) knots 0 0 0 1 1 1
  spline S484 degree 2 poles (4.4378, -4.1091) (4.5824, -3.9918) (4.8006, -3.9918) knots 0 0 0 1 1 1
  spline S485 degree 2 poles (4.8006, -3.9918) (4.9616, -3.9918) (5.083, -4.0573) knots 0 0 0 1 1 1
  spline S486 degree 2 poles (5.083, -4.0573) (5.2045, -4.1214) (5.2836, -4.2442) knots 0 0 0 1 1 1
  spline S487 degree 2 poles (5.2836, -4.2442) (5.3627, -4.3656) (5.4077, -4.5416) knots 0 0 0 1 1 1
  spline S488 degree 2 poles (5.4077, -4.5416) (5.4528, -4.7162) (5.4528, -5.0136) knots 0 0 0 1 1 1
  spline S489 degree 2 poles (5.4528, -5.0136) (5.4528, -5.3656) (5.3805, -5.5825) knots 0 0 0 1 1 1
  spline S490 degree 2 poles (5.3805, -5.5825) (5.3082, -5.7981) (5.1635, -5.9168) knots 0 0 0 1 1 1
  spline S491 degree 2 poles (5.1635, -5.9168) (5.0203, -6.0341) (4.8006, -6.0341) knots 0 0 0 1 1 1
  spline S492 degree 2 poles (4.8006, -6.0341) (4.5114, -6.0341) (4.3464, -5.8267) knots 0 0 0 1 1 1
  spline S493 degree 2 poles (4.3464, -5.8267) (4.1485, -5.5771) (4.1485, -5.0136) knots 0 0 0 1 1 1
  spline S494 degree 2 poles (4.4009, -5.0136) (4.4009, -5.5061) (4.5155, -5.6698) knots 0 0 0 1 1 1
  spline S495 degree 2 poles (4.5155, -5.6698) (4.6315, -5.8322) (4.8006, -5.8322) knots 0 0 0 1 1 1
  spline S496 degree 2 poles (4.8006, -5.8322) (4.9698, -5.8322) (5.0844, -5.6685) knots 0 0 0 1 1 1
  spline S497 degree 2 poles (5.0844, -5.6685) (5.2004, -5.5048) (5.2004, -5.0136) knots 0 0 0 1 1 1
  spline S498 degree 2 poles (5.2004, -5.0136) (5.2004, -4.5198) (5.0844, -4.3574) knots 0 0 0 1 1 1
  spline S499 degree 2 poles (5.0844, -4.3574) (4.9698, -4.1951) (4.7979, -4.1951) knots 0 0 0 1 1 1
  spline S500 degree 2 poles (4.7979, -4.1951) (4.6288, -4.1951) (4.5278, -4.3383) knots 0 0 0 1 1 1
  spline S501 degree 2 poles (4.5278, -4.3383) (4.4009, -4.5211) (4.4009, -5.0136) knots 0 0 0 1 1 1
  line L266 (6.3736, -6) -> (5.5987, -4)
  line L267 (5.5987, -4) -> (5.8852, -4)
  line L268 (5.8852, -4) -> (6.405, -5.4529)
  spline S502 degree 2 poles (6.405, -5.4529) (6.4678, -5.6276) (6.5101, -5.7804) knots 0 0 0 1 1 1
  spline S503 degree 2 poles (6.5101, -5.7804) (6.5564, -5.6166) (6.6178, -5.4529) knots 0 0 0 1 1 1
  line L269 (6.6178, -5.4529) -> (7.1581, -4)
  line L270 (7.1581, -4) -> (7.4282, -4)
  line L271 (7.4282, -4) -> (6.6451, -6)
  line L272 (6.6451, -6) -> (6.3736, -6)
  line L273 (7.6656, -6) -> (7.6656, -4)
  line L274 (7.6656, -4) -> (8.3545, -4)
  spline S504 degree 2 poles (8.3545, -4) (8.5878, -4) (8.7106, -4.0286) knots 0 0 0 1 1 1
  spline S505 degree 2 poles (8.7106, -4.0286) (8.8825, -4.0682) (9.0039, -4.1719) knots 0 0 0 1 1 1
  spline S506 degree 2 poles (9.0039, -4.1719) (9.1622, -4.3056) (9.2399, -4.5143) knots 0 0 0 1 1 1
  spline S507 degree 2 poles (9.2399, -4.5143) (9.3191, -4.7217) (9.3191, -4.9891) knots 0 0 0 1 1 1
  spline S508 degree 2 poles (9.3191, -4.9891) (9.3191, -5.2169) (9.2659, -5.3929) knots 0 0 0 1 1 1
  spline S509 degree 2 poles (9.2659, -5.3929) (9.2127, -5.5689) (9.1294, -5.6849) knots 0 0 0 1 1 1
  spline S510 degree 2 poles (9.1294, -5.6849) (9.0462, -5.7995) (8.9466, -5.8663) knots 0 0 0 1 1 1
  spline S511 degree 2 poles (8.9466, -5.8663) (8.8484, -5.9318) (8.7079, -5.9659) knots 0 0 0 1 1 1
  spline S512 degree 2 poles (8.7079, -5.9659) (8.5687, -6) (8.3873, -6) knots 0 0 0 1 1 1
  line L275 (8.3873, -6) -> (7.6656, -6)
  line L276 (7.9303, -5.764) -> (8.3573, -5.764)
  spline S513 degree 2 poles (8.3573, -5.764) (8.5551, -5.764) (8.667, -5.7271) knots 0 0 0 1 1 1
  spline S514 degree 2 poles (8.667, -5.7271) (8.7802, -5.6903) (8.847, -5.6235) knots 0 0 0 1 1 1
  spline S515 degree 2 poles (8.847, -5.6235) (8.9412, -5.5293) (8.993, -5.3711) knots 0 0 0 1 1 1
  spline S516 degree 2 poles (8.993, -5.3711) (9.0462, -5.2115) (9.0462, -4.985) knots 0 0 0 1 1 1
  spline S517 degree 2 poles (9.0462, -4.985) (9.0462, -4.6712) (8.9425, -4.5034) knots 0 0 0 1 1 1
  spline S518 degree 2 poles (8.9425, -4.5034) (8.8402, -4.3342) (8.6929, -4.2769) knots 0 0 0 1 1 1
  spline S519 degree 2 poles (8.6929, -4.2769) (8.5865, -4.236) (8.3504, -4.236) knots 0 0 0 1 1 1
  line L277 (8.3504, -4.236) -> (7.9303, -4.236)
  line L278 (7.9303, -4.236) -> (7.9303, -5.764)
  line L279 (11.1103, -5.2988) -> (11.375, -5.3656)
  spline S520 degree 2 poles (11.375, -5.3656) (11.2918, -5.6917) (11.0749, -5.8636) knots 0 0 0 1 1 1
  spline S521 degree 2 poles (11.0749, -5.8636) (10.8593, -6.0341) (10.5469, -6.0341) knots 0 0 0 1 1 1
  spline S522 degree 2 poles (10.5469, -6.0341) (10.2236, -6.0341) (10.0203, -5.9031) knots 0 0 0 1 1 1
  spline S523 degree 2 poles (10.0203, -5.9031) (9.8184, -5.7708) (9.712, -5.5211) knots 0 0 0 1 1 1
  spline S524 degree 2 poles (9.712, -5.5211) (9.6069, -5.2715) (9.6069, -4.985) knots 0 0 0 1 1 1
  spline S525 degree 2 poles (9.6069, -4.985) (9.6069, -4.6726) (9.7256, -4.4407) knots 0 0 0 1 1 1
  spline S526 degree 2 poles (9.7256, -4.4407) (9.8457, -4.2074) (10.0653, -4.0873) knots 0 0 0 1 1 1
  spline S527 degree 2 poles (10.0653, -4.0873) (10.2863, -3.9659) (10.551, -3.9659) knots 0 0 0 1 1 1
  spline S528 degree 2 poles (10.551, -3.9659) (10.8511, -3.9659) (11.0558, -4.1187) knots 0 0 0 1 1 1
  spline S529 degree 2 poles (11.0558, -4.1187) (11.2604, -4.2715) (11.3409, -4.5484) knots 0 0 0 1 1 1
  line L280 (11.3409, -4.5484) -> (11.0803, -4.6098)
  spline S530 degree 2 poles (11.0803, -4.6098) (11.0107, -4.3915) (10.8784, -4.292) knots 0 0 0 1 1 1
  spline S531 degree 2 poles (10.8784, -4.292) (10.7461, -4.1924) (10.5455, -4.1924) knots 0 0 0 1 1 1
  spline S532 degree 2 poles (10.5455, -4.1924) (10.315, -4.1924) (10.1594, -4.3029) knots 0 0 0 1 1 1
  spline S533 degree 2 poles (10.1594, -4.3029) (10.0053, -4.4134) (9.9425, -4.6003) knots 0 0 0 1 1 1
  spline S534 degree 2 poles (9.9425, -4.6003) (9.8798, -4.7858) (9.8798, -4.9836) knots 0 0 0 1 1 1
  spline S535 degree 2 poles (9.8798, -4.9836) (9.8798, -5.2387) (9.9534, -5.4297) knots 0 0 0 1 1 1
  spline S536 degree 2 poles (9.9534, -5.4297) (10.0285, -5.6194) (10.1854, -5.7135) knots 0 0 0 1 1 1
  spline S537 degree 2 poles (10.1854, -5.7135) (10.3423, -5.8076) (10.5251, -5.8076) knots 0 0 0 1 1 1
  spline S538 degree 2 poles (10.5251, -5.8076) (10.7474, -5.8076) (10.9016, -5.6794) knots 0 0 0 1 1 1
  spline S539 degree 2 poles (10.9016, -5.6794) (11.0558, -5.5512) (11.1103, -5.2988) knots 0 0 0 1 1 1
  spline S540 degree 2 poles (-11.2539, 3.9898) (-11.2539, 4.2558) (-11.1997, 4.4175) knots 0 0 0 1 1 1
  spline S541 degree 2 poles (-11.1997, 4.4175) (-11.1444, 4.5802) (-11.037, 4.6681) knots 0 0 0 1 1 1
  spline S542 degree 2 poles (-11.037, 4.6681) (-10.9285, 4.7561) (-10.7648, 4.7561) knots 0 0 0 1 1 1
  spline S543 degree 2 poles (-10.7648, 4.7561) (-10.6441, 4.7561) (-10.553, 4.707) knots 0 0 0 1 1 1
  spline S544 degree 2 poles (-10.553, 4.707) (-10.4619, 4.6589) (-10.4026, 4.5668) knots 0 0 0 1 1 1
  spline S545 degree 2 poles (-10.4026, 4.5668) (-10.3432, 4.4758) (-10.3095, 4.3438) knots 0 0 0 1 1 1
  spline S546 degree 2 poles (-10.3095, 4.3438) (-10.2757, 4.2128) (-10.2757, 3.9898) knots 0 0 0 1 1 1
  spline S547 degree 2 poles (-10.2757, 3.9898) (-10.2757, 3.7258) (-10.3299, 3.5631) knots 0 0 0 1 1 1
  spline S548 degree 2 poles (-10.3299, 3.5631) (-10.3842, 3.4014) (-10.4926, 3.3124) knots 0 0 0 1 1 1
  spline S549 degree 2 poles (-10.4926, 3.3124) (-10.6001, 3.2244) (-10.7648, 3.2244) knots 0 0 0 1 1 1
  spline S550 degree 2 poles (-10.7648, 3.2244) (-10.9817, 3.2244) (-11.1055, 3.3799) knots 0 0 0 1 1 1
  spline S551 degree 2 poles (-11.1055, 3.3799) (-11.2539, 3.5672) (-11.2539, 3.9898) knots 0 0 0 1 1 1
  spline S552 degree 2 poles (-11.0646, 3.9898) (-11.0646, 3.6204) (-10.9787, 3.4976) knots 0 0 0 1 1 1
  spline S553 degree 2 poles (-10.9787, 3.4976) (-10.8917, 3.3759) (-10.7648, 3.3759) knots 0 0 0 1 1 1
  spline S554 degree 2 poles (-10.7648, 3.3759) (-10.6379, 3.3759) (-10.552, 3.4986) knots 0 0 0 1 1 1
  spline S555 degree 2 poles (-10.552, 3.4986) (-10.465, 3.6214) (-10.465, 3.9898) knots 0 0 0 1 1 1
  spline S556 degree 2 poles (-10.465, 3.9898) (-10.465, 4.3602) (-10.552, 4.4819) knots 0 0 0 1 1 1
  spline S557 degree 2 poles (-10.552, 4.4819) (-10.6379, 4.6037) (-10.7669, 4.6037) knots 0 0 0 1 1 1
  spline S558 degree 2 poles (-10.7669, 4.6037) (-10.8937, 4.6037) (-10.9694, 4.4962) knots 0 0 0 1 1 1
  spline S559 degree 2 poles (-10.9694, 4.4962) (-11.0646, 4.3591) (-11.0646, 3.9898) knots 0 0 0 1 1 1
  line L281 (-10.0875, 3.646) -> (-9.9033, 3.6705)
  spline S560 degree 2 poles (-9.9033, 3.6705) (-9.8716, 3.514) (-9.7958, 3.4444) knots 0 0 0 1 1 1
  spline S561 degree 2 poles (-9.7958, 3.4444) (-9.7191, 3.3759) (-9.6096, 3.3759) knots 0 0 0 1 1 1
  spline S562 degree 2 poles (-9.6096, 3.3759) (-9.4797, 3.3759) (-9.3907, 3.4659) knots 0 0 0 1 1 1
  spline S563 degree 2 poles (-9.3907, 3.4659) (-9.3006, 3.5559) (-9.3006, 3.6889) knots 0 0 0 1 1 1
  spline S564 degree 2 poles (-9.3006, 3.6889) (-9.3006, 3.8158) (-9.3835, 3.8977) knots 0 0 0 1 1 1
  spline S565 degree 2 poles (-9.3835, 3.8977) (-9.4664, 3.9806) (-9.5943, 3.9806) knots 0 0 0 1 1 1
  spline S566 degree 2 poles (-9.5943, 3.9806) (-9.6465, 3.9806) (-9.7242, 3.9601) knots 0 0 0 1 1 1
  line L282 (-9.7242, 3.9601) -> (-9.7038, 4.1218)
  spline S567 degree 2 poles (-9.7038, 4.1218) (-9.6853, 4.1197) (-9.6741, 4.1197) knots 0 0 0 1 1 1
  spline S568 degree 2 poles (-9.6741, 4.1197) (-9.5564, 4.1197) (-9.4623, 4.1811) knots 0 0 0 1 1 1
  spline S569 degree 2 poles (-9.4623, 4.1811) (-9.3681, 4.2425) (-9.3681, 4.3704) knots 0 0 0 1 1 1
  spline S570 degree 2 poles (-9.3681, 4.3704) (-9.3681, 4.4717) (-9.4367, 4.5382) knots 0 0 0 1 1 1
  spline S571 degree 2 poles (-9.4367, 4.5382) (-9.5053, 4.6047) (-9.6137, 4.6047) knots 0 0 0 1 1 1
  spline S572 degree 2 poles (-9.6137, 4.6047) (-9.7211, 4.6047) (-9.7928, 4.5372) knots 0 0 0 1 1 1
  spline S573 degree 2 poles (-9.7928, 4.5372) (-9.8644, 4.4696) (-9.8849, 4.3346) knots 0 0 0 1 1 1
  line L283 (-9.8849, 4.3346) -> (-10.069, 4.3673)
  spline S574 degree 2 poles (-10.069, 4.3673) (-10.0353, 4.5525) (-9.9156, 4.6538) knots 0 0 0 1 1 1
  spline S575 degree 2 poles (-9.9156, 4.6538) (-9.7958, 4.7561) (-9.6178, 4.7561) knots 0 0 0 1 1 1
  spline S576 degree 2 poles (-9.6178, 4.7561) (-9.495, 4.7561) (-9.3917, 4.7029) knots 0 0 0 1 1 1
  spline S577 degree 2 poles (-9.3917, 4.7029) (-9.2883, 4.6508) (-9.2341, 4.5597) knots 0 0 0 1 1 1
  spline S578 degree 2 poles (-9.2341, 4.5597) (-9.1789, 4.4686) (-9.1789, 4.3663) knots 0 0 0 1 1 1
  spline S579 degree 2 poles (-9.1789, 4.3663) (-9.1789, 4.2691) (-9.231, 4.1893) knots 0 0 0 1 1 1
  spline S580 degree 2 poles (-9.231, 4.1893) (-9.2832, 4.1095) (-9.3855, 4.0624) knots 0 0 0 1 1 1
  spline S581 degree 2 poles (-9.3855, 4.0624) (-9.2525, 4.0317) (-9.1789, 3.9345) knots 0 0 0 1 1 1
  spline S582 degree 2 poles (-9.1789, 3.9345) (-9.1052, 3.8383) (-9.1052, 3.693) knots 0 0 0 1 1 1
  spline S583 degree 2 poles (-9.1052, 3.693) (-9.1052, 3.4966) (-9.2484, 3.3595) knots 0 0 0 1 1 1
  spline S584 degree 2 poles (-9.2484, 3.3595) (-9.3917, 3.2234) (-9.6106, 3.2234) knots 0 0 0 1 1 1
  spline S585 degree 2 poles (-9.6106, 3.2234) (-9.8081, 3.2234) (-9.9391, 3.3411) knots 0 0 0 1 1 1
  spline S586 degree 2 poles (-9.9391, 3.3411) (-10.069, 3.4587) (-10.0875, 3.646) knots 0 0 0 1 1 1
  line L284 (-7.9551, 3.427) -> (-7.9551, 3.25)
  line L285 (-7.9551, 3.25) -> (-8.9466, 3.25)
  spline S587 degree 2 poles (-8.9466, 3.25) (-8.9486, 3.3165) (-8.9251, 3.3779) knots 0 0 0 1 1 1
  spline S588 degree 2 poles (-8.9251, 3.3779) (-8.8872, 3.4792) (-8.8044, 3.5774) knots 0 0 0 1 1 1
  spline S589 degree 2 poles (-8.8044, 3.5774) (-8.7205, 3.6756) (-8.5629, 3.8046) knots 0 0 0 1 1 1
  spline S590 degree 2 poles (-8.5629, 3.8046) (-8.3184, 4.0051) (-8.2324, 4.1218) knots 0 0 0 1 1 1
  spline S591 degree 2 poles (-8.2324, 4.1218) (-8.1465, 4.2394) (-8.1465, 4.3438) knots 0 0 0 1 1 1
  spline S592 degree 2 poles (-8.1465, 4.3438) (-8.1465, 4.4533) (-8.2252, 4.528) knots 0 0 0 1 1 1
  spline S593 degree 2 poles (-8.2252, 4.528) (-8.303, 4.6037) (-8.4289, 4.6037) knots 0 0 0 1 1 1
  spline S594 degree 2 poles (-8.4289, 4.6037) (-8.5619, 4.6037) (-8.6417, 4.5239) knots 0 0 0 1 1 1
  spline S595 degree 2 poles (-8.6417, 4.5239) (-8.7215, 4.4441) (-8.7225, 4.3029) knots 0 0 0 1 1 1
  line L286 (-8.7225, 4.3029) -> (-8.9118, 4.3223)
  spline S596 degree 2 poles (-8.9118, 4.3223) (-8.8924, 4.5341) (-8.7655, 4.6446) knots 0 0 0 1 1 1
  spline S597 degree 2 poles (-8.7655, 4.6446) (-8.6386, 4.7561) (-8.4248, 4.7561) knots 0 0 0 1 1 1
  spline S598 degree 2 poles (-8.4248, 4.7561) (-8.2089, 4.7561) (-8.083, 4.6364) knots 0 0 0 1 1 1
  spline S599 degree 2 poles (-8.083, 4.6364) (-7.9572, 4.5167) (-7.9572, 4.3397) knots 0 0 0 1 1 1
  spline S600 degree 2 poles (-7.9572, 4.3397) (-7.9572, 4.2497) (-7.994, 4.1627) knots 0 0 0 1 1 1
  spline S601 degree 2 poles (-7.994, 4.1627) (-8.0308, 4.0757) (-8.1168, 3.9795) knots 0 0 0 1 1 1
  spline S602 degree 2 poles (-8.1168, 3.9795) (-8.2017, 3.8834) (-8.4002, 3.7156) knots 0 0 0 1 1 1
  spline S603 degree 2 poles (-8.4002, 3.7156) (-8.566, 3.5764) (-8.613, 3.5263) knots 0 0 0 1 1 1
  spline S604 degree 2 poles (-8.613, 3.5263) (-8.6601, 3.4771) (-8.6908, 3.427) knots 0 0 0 1 1 1
  line L287 (-8.6908, 3.427) -> (-7.9551, 3.427)
  line L288 (-7.7566, 3.646) -> (-7.5724, 3.6705)
  spline S605 degree 2 poles (-7.5724, 3.6705) (-7.5407, 3.514) (-7.465, 3.4444) knots 0 0 0 1 1 1
  spline S606 degree 2 poles (-7.465, 3.4444) (-7.3883, 3.3759) (-7.2788, 3.3759) knots 0 0 0 1 1 1
  spline S607 degree 2 poles (-7.2788, 3.3759) (-7.1488, 3.3759) (-7.0598, 3.4659) knots 0 0 0 1 1 1
  spline S608 degree 2 poles (-7.0598, 3.4659) (-6.9698, 3.5559) (-6.9698, 3.6889) knots 0 0 0 1 1 1
  spline S609 degree 2 poles (-6.9698, 3.6889) (-6.9698, 3.8158) (-7.0527, 3.8977) knots 0 0 0 1 1 1
  spline S610 degree 2 poles (-7.0527, 3.8977) (-7.1355, 3.9806) (-7.2634, 3.9806) knots 0 0 0 1 1 1
  spline S611 degree 2 poles (-7.2634, 3.9806) (-7.3156, 3.9806) (-7.3934, 3.9601) knots 0 0 0 1 1 1
  line L289 (-7.3934, 3.9601) -> (-7.3729, 4.1218)
  spline S612 degree 2 poles (-7.3729, 4.1218) (-7.3545, 4.1197) (-7.3432, 4.1197) knots 0 0 0 1 1 1
  spline S613 degree 2 poles (-7.3432, 4.1197) (-7.2256, 4.1197) (-7.1314, 4.1811) knots 0 0 0 1 1 1
  spline S614 degree 2 poles (-7.1314, 4.1811) (-7.0373, 4.2425) (-7.0373, 4.3704) knots 0 0 0 1 1 1
  spline S615 degree 2 poles (-7.0373, 4.3704) (-7.0373, 4.4717) (-7.1059, 4.5382) knots 0 0 0 1 1 1
  spline S616 degree 2 poles (-7.1059, 4.5382) (-7.1744, 4.6047) (-7.2829, 4.6047) knots 0 0 0 1 1 1
  spline S617 degree 2 poles (-7.2829, 4.6047) (-7.3903, 4.6047) (-7.4619, 4.5372) knots 0 0 0 1 1 1
  spline S618 degree 2 poles (-7.4619, 4.5372) (-7.5336, 4.4696) (-7.554, 4.3346) knots 0 0 0 1 1 1
  line L290 (-7.554, 4.3346) -> (-7.7382, 4.3673)
  spline S619 degree 2 poles (-7.7382, 4.3673) (-7.7044, 4.5525) (-7.5847, 4.6538) knots 0 0 0 1 1 1
  spline S620 degree 2 poles (-7.5847, 4.6538) (-7.465, 4.7561) (-7.287, 4.7561) knots 0 0 0 1 1 1